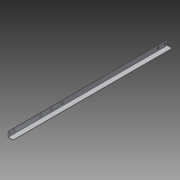
# Autodesk Inventor part: Shooter Side Support Bar - R
Saved by Autodesk Inventor 2014 SP1 (Build 180222100, 222)
## iProperties
Created: 2013-12-13
Part Number: Shooter Side Support Bar - R
Material: Aluminum 6061
Document SubType Name: Modeling
Designer: Moses
Mass: 32.4416 g
Surface Area: 311.167 cm^2
Volume: 11.9711 cm^3
Density: 2.71 g/cm^3
Appearance: Aluminum - Flat
Author: Moses
Autodesk Inventor part; units mm, degrees
ref_plane "YZ Plane" through (0, 0, 0) normal (1, 0, 0) x (0, 1, 0)
ref_plane "XZ Plane" through (0, 0, 0) normal (0, 1, 0) x (-1, 0, 0)
ref_plane "XY Plane" through (0, 0, 0) normal (0, 0, 1) x (1, 0, 0)
sketch "Sketch1" plane through (0, 0, 0) normal (0, 0, 1) x (1, 0, 0)
  line L0 (0, 0) -> (0, 15.875)
  line L1 (0, 15.875) -> (0.7937, 15.875)
  line L2 (0.7937, 15.875) -> (0.7938, 0.7937)
  line L3 (0.7938, 0.7937) -> (15.875, 0.7937)
  line L4 (15.875, 0.7937) -> (15.875, 0)
  line L5 (15.875, 0) -> (0, 0)
  dimension "d0" = 15.875
  dimension "d1" = 0.7937
  constraints: 12 end point, 3 horizontal, 3 vertical, 2 perpendicular
  measures "d0" distance of L0.start L0.end
  measures "d1" distance of L0.end L1.end
extrude "Extrusion1" add sketch "Sketch1" along normal blind 495.3
sketch "Sketch2" plane through (0, 0, 0) normal (-1, 0, 0) x (0, 0, 1)
  line L0 (276.0218, 396.0812) -> (276.0218, 91.2812) projected
  arc A0 (276.0218, 91.2812) -> (282.7782, 91.2812) centre (279.4, 91.2812) ccw projected
  line L1 (282.7782, 91.2812) -> (282.7782, 396.0812) projected
  arc A1 (282.7782, 396.0812) -> (276.0218, 396.0812) centre (279.4, 396.0812) ccw projected
  circle A2 centre (279.4, 27.7812) radius 3.3782 projected
  circle A3 centre (279.4, 59.5312) radius 3.3782 projected
  line L2 (292.1, 15.0812) -> (482.6, 15.0812) projected
  line L3 (482.6, 15.0812) -> (482.6, 484.9812) projected
  line L4 (482.6, 484.9812) -> (292.1, 484.9812) projected
  line L5 (292.1, 484.9812) -> (292.1, 15.0812) projected
  line L6 (149.0218, 396.0812) -> (149.0218, 91.2812) projected
  arc A4 (149.0218, 91.2812) -> (155.7782, 91.2812) centre (152.4, 91.2812) ccw projected
  line L7 (155.7782, 91.2812) -> (155.7782, 396.0812) projected
  arc A5 (155.7782, 396.0812) -> (149.0218, 396.0812) centre (152.4, 396.0812) ccw projected
  ellipse E0 centre (152.3984, 27.7812) end of major axis (152.3984, 31.1594) minor radius 3.3782 projected
  ellipse E1 centre (152.3984, 59.5312) end of major axis (152.3984, 56.153) minor radius 3.3782 projected
  line L8 (266.7, 15.0812) -> (266.7, 484.9812) projected
  line L9 (266.7, 484.9812) -> (165.1, 484.9812) projected
  line L10 (165.1, 484.9812) -> (165.1, 15.0812) projected
  line L11 (165.1, 15.0812) -> (266.7, 15.0812) projected
  line L12 (12.7, 15.0812) -> (139.7, 15.0812) projected
  line L13 (139.7, 15.0812) -> (139.7, 484.9812) projected
  line L14 (139.7, 484.9812) -> (12.7, 484.9812) projected
  line L15 (12.7, 484.9812) -> (12.7, 15.0812) projected
  circle A6 centre (393.7, 8.7312) radius 3.3782 projected
  circle A7 centre (393.7, 491.3312) radius 3.3782 projected
  circle A8 centre (405.6062, 8.7312) radius 3.3782 projected
  circle A9 centre (405.6062, 491.3312) radius 3.3782 projected
  circle A10 centre (417.5125, 8.7312) radius 3.3782 projected
  circle A11 centre (417.5125, 491.3312) radius 3.3782 projected
  circle A12 centre (429.4187, 8.7312) radius 3.3782 projected
  circle A13 centre (429.4187, 491.3312) radius 3.3782 projected
  circle A14 centre (441.325, 8.7312) radius 3.3782 projected
  circle A15 centre (441.325, 491.3312) radius 3.3782 projected
  circle A16 centre (453.2312, 8.7312) radius 3.3782 projected
  circle A17 centre (453.2312, 491.3312) radius 3.3782 projected
  circle A18 centre (465.1375, 8.7312) radius 3.3782 projected
  circle A19 centre (465.1375, 491.3312) radius 3.3782 projected
  circle A20 centre (477.0437, 8.7312) radius 3.3782 projected
  circle A21 centre (477.0437, 491.3312) radius 3.3782 projected
  circle A22 centre (382.6329, 8.7312) radius 3.3782 projected
  circle A23 centre (382.6329, 491.3312) radius 3.3782 projected
  circle A24 centre (371.5657, 8.7312) radius 3.3782 projected
  circle A25 centre (371.5657, 491.3312) radius 3.3782 projected
  circle A26 centre (360.4986, 8.7312) radius 3.3782 projected
  circle A27 centre (360.4986, 491.3312) radius 3.3782 projected
  circle A28 centre (349.4314, 8.7312) radius 3.3782 projected
  circle A29 centre (349.4314, 491.3312) radius 3.3782 projected
  circle A30 centre (338.3643, 8.7312) radius 3.3782 projected
  circle A31 centre (338.3643, 491.3312) radius 3.3782 projected
  circle A32 centre (327.2971, 8.7312) radius 3.3782 projected
  circle A33 centre (327.2971, 491.3312) radius 3.3782 projected
  circle A34 centre (316.23, 8.7312) radius 3.3782 projected
  circle A35 centre (316.23, 491.3312) radius 3.3782 projected
  circle A36 centre (305.1629, 8.7312) radius 3.3782 projected
  circle A37 centre (305.1629, 491.3312) radius 3.3782 projected
  circle A38 centre (294.0957, 8.7312) radius 3.3782 projected
  circle A39 centre (294.0957, 491.3312) radius 3.3782 projected
  circle A40 centre (283.0286, 8.7312) radius 3.3782 projected
  circle A41 centre (283.0286, 491.3312) radius 3.3782 projected
  circle A42 centre (271.9614, 8.7312) radius 3.3782 projected
  circle A43 centre (271.9614, 491.3312) radius 3.3782 projected
  circle A44 centre (260.8943, 8.7312) radius 3.3782 projected
  circle A45 centre (260.8943, 491.3312) radius 3.3782 projected
  circle A46 centre (249.8271, 8.7312) radius 3.3782 projected
  circle A47 centre (249.8271, 491.3312) radius 3.3782 projected
  circle A48 centre (238.76, 8.7312) radius 3.3782 projected
  circle A49 centre (238.76, 491.3312) radius 3.3782 projected
  circle A50 centre (227.6929, 8.7312) radius 3.3782 projected
  circle A51 centre (227.6929, 491.3312) radius 3.3782 projected
  circle A52 centre (216.6257, 8.7312) radius 3.3782 projected
  circle A53 centre (216.6257, 491.3312) radius 3.3782 projected
  circle A54 centre (205.5586, 8.7312) radius 3.3782 projected
  circle A55 centre (205.5586, 491.3312) radius 3.3782 projected
  circle A56 centre (194.4914, 8.7312) radius 3.3782 projected
  circle A57 centre (194.4914, 491.3312) radius 3.3782 projected
  circle A58 centre (183.4243, 8.7312) radius 3.3782 projected
  circle A59 centre (183.4243, 491.3312) radius 3.3782 projected
  circle A60 centre (172.3571, 8.7312) radius 3.3782 projected
  circle A61 centre (172.3571, 491.3312) radius 3.3782 projected
  circle A62 centre (161.29, 8.7312) radius 3.3782 projected
  circle A63 centre (161.29, 491.3312) radius 3.3782 projected
  circle A64 centre (150.2229, 8.7312) radius 3.3782 projected
  circle A65 centre (150.2229, 491.3312) radius 3.3782 projected
  circle A66 centre (139.1557, 8.7312) radius 3.3782 projected
  circle A67 centre (139.1557, 491.3312) radius 3.3782 projected
  circle A68 centre (128.0886, 8.7312) radius 3.3782 projected
  circle A69 centre (128.0886, 491.3312) radius 3.3782 projected
  circle A70 centre (117.0214, 8.7312) radius 3.3782 projected
  circle A71 centre (117.0214, 491.3312) radius 3.3782 projected
  circle A72 centre (105.9543, 8.7312) radius 3.3782 projected
  circle A73 centre (105.9543, 491.3312) radius 3.3782 projected
  circle A74 centre (94.8871, 8.7312) radius 3.3782 projected
  circle A75 centre (94.8871, 491.3312) radius 3.3782 projected
  circle A76 centre (83.82, 8.7312) radius 3.3782 projected
  circle A77 centre (83.82, 491.3312) radius 3.3782 projected
  circle A78 centre (72.7529, 8.7312) radius 3.3782 projected
  circle A79 centre (72.7529, 491.3312) radius 3.3782 projected
  circle A80 centre (61.6857, 8.7312) radius 3.3782 projected
  circle A81 centre (61.6857, 491.3312) radius 3.3782 projected
  circle A82 centre (50.6186, 8.7312) radius 3.3782 projected
  circle A83 centre (50.6186, 491.3312) radius 3.3782 projected
  circle A84 centre (39.5514, 8.7312) radius 3.3782 projected
  circle A85 centre (39.5514, 491.3312) radius 3.3782 projected
  circle A86 centre (28.4843, 8.7312) radius 3.3782 projected
  circle A87 centre (28.4843, 491.3312) radius 3.3782 projected
  circle A88 centre (17.4171, 8.7312) radius 3.3782 projected
  circle A89 centre (17.4171, 491.3312) radius 3.3782 projected
  circle A90 centre (488.95, 8.7312) radius 3.3782 projected
  circle A91 centre (488.95, 18.5802) radius 3.3782 projected
  circle A92 centre (488.95, 28.4292) radius 3.3782 projected
  circle A93 centre (488.95, 38.2782) radius 3.3782 projected
  circle A94 centre (488.95, 48.1272) radius 3.3782 projected
  circle A95 centre (488.95, 57.9761) radius 3.3782 projected
  circle A96 centre (488.95, 67.8251) radius 3.3782 projected
  circle A97 centre (488.95, 77.6741) radius 3.3782 projected
  circle A98 centre (488.95, 87.5231) radius 3.3782 projected
  circle A99 centre (488.95, 97.3721) radius 3.3782 projected
  circle A100 centre (488.95, 107.221) radius 3.3782 projected
  circle A101 centre (488.95, 117.07) radius 3.3782 projected
  circle A102 centre (488.95, 126.919) radius 3.3782 projected
  circle A103 centre (488.95, 136.768) radius 3.3782 projected
  circle A104 centre (488.95, 146.617) radius 3.3782 projected
  circle A105 centre (488.95, 156.4659) radius 3.3782 projected
  circle A106 centre (488.95, 166.3149) radius 3.3782 projected
  circle A107 centre (488.95, 176.1639) radius 3.3782 projected
  circle A108 centre (488.95, 186.0129) radius 3.3782 projected
  circle A109 centre (488.95, 195.8619) radius 3.3782 projected
  circle A110 centre (488.95, 205.7108) radius 3.3782 projected
  circle A111 centre (488.95, 215.5598) radius 3.3782 projected
  circle A112 centre (488.95, 225.4088) radius 3.3782 projected
  circle A113 centre (488.95, 235.2578) radius 3.3782 projected
  circle A114 centre (488.95, 245.1068) radius 3.3782 projected
  circle A115 centre (488.95, 254.9557) radius 3.3782 projected
  circle A116 centre (488.95, 264.8047) radius 3.3782 projected
  circle A117 centre (488.95, 274.6537) radius 3.3782 projected
  circle A118 centre (488.95, 284.5027) radius 3.3782 projected
  circle A119 centre (488.95, 294.3517) radius 3.3782 projected
  circle A120 centre (488.95, 304.2006) radius 3.3782 projected
  circle A121 centre (488.95, 314.0496) radius 3.3782 projected
  circle A122 centre (488.95, 323.8986) radius 3.3782 projected
  circle A123 centre (488.95, 333.7476) radius 3.3782 projected
  circle A124 centre (488.95, 343.5966) radius 3.3782 projected
  circle A125 centre (488.95, 353.4455) radius 3.3782 projected
  circle A126 centre (488.95, 363.2945) radius 3.3782 projected
  circle A127 centre (488.95, 373.1435) radius 3.3782 projected
  circle A128 centre (488.95, 382.9925) radius 3.3782 projected
  circle A129 centre (488.95, 392.8415) radius 3.3782 projected
  circle A130 centre (488.95, 402.6904) radius 3.3782 projected
  circle A131 centre (488.95, 412.5394) radius 3.3782 projected
  circle A132 centre (488.95, 422.3884) radius 3.3782 projected
  circle A133 centre (488.95, 432.2374) radius 3.3782 projected
  circle A134 centre (488.95, 442.0864) radius 3.3782 projected
  circle A135 centre (488.95, 451.9353) radius 3.3782 projected
  circle A136 centre (488.95, 461.7843) radius 3.3782 projected
  circle A137 centre (488.95, 471.6333) radius 3.3782 projected
  circle A138 centre (488.95, 481.4823) radius 3.3782 projected
  circle A139 centre (488.95, 491.3312) radius 3.3782 projected
  circle A140 centre (6.35, 8.7312) radius 3.3782 projected
  circle A141 centre (6.35, 18.5802) radius 3.3782 projected
  circle A142 centre (6.35, 28.4292) radius 3.3782 projected
  circle A143 centre (6.35, 38.2782) radius 3.3782 projected
  circle A144 centre (6.35, 48.1272) radius 3.3782 projected
  circle A145 centre (6.35, 57.9761) radius 3.3782 projected
  circle A146 centre (6.35, 67.8251) radius 3.3782 projected
  circle A147 centre (6.35, 77.6741) radius 3.3782 projected
  circle A148 centre (6.35, 87.5231) radius 3.3782 projected
  circle A149 centre (6.35, 97.3721) radius 3.3782 projected
  circle A150 centre (6.35, 107.221) radius 3.3782 projected
  circle A151 centre (6.35, 117.07) radius 3.3782 projected
  circle A152 centre (6.35, 126.919) radius 3.3782 projected
  circle A153 centre (6.35, 136.768) radius 3.3782 projected
  circle A154 centre (6.35, 146.617) radius 3.3782 projected
  circle A155 centre (6.35, 156.4659) radius 3.3782 projected
  circle A156 centre (6.35, 166.3149) radius 3.3782 projected
  circle A157 centre (6.35, 176.1639) radius 3.3782 projected
  circle A158 centre (6.35, 186.0129) radius 3.3782 projected
  circle A159 centre (6.35, 195.8619) radius 3.3782 projected
  circle A160 centre (6.35, 205.7108) radius 3.3782 projected
  circle A161 centre (6.35, 215.5598) radius 3.3782 projected
  circle A162 centre (6.35, 225.4088) radius 3.3782 projected
  circle A163 centre (6.35, 235.2578) radius 3.3782 projected
  circle A164 centre (6.35, 245.1068) radius 3.3782 projected
  circle A165 centre (6.35, 254.9557) radius 3.3782 projected
  circle A166 centre (6.35, 264.8047) radius 3.3782 projected
  circle A167 centre (6.35, 274.6537) radius 3.3782 projected
  circle A168 centre (6.35, 284.5027) radius 3.3782 projected
  circle A169 centre (6.35, 294.3517) radius 3.3782 projected
  circle A170 centre (6.35, 304.2006) radius 3.3782 projected
  circle A171 centre (6.35, 314.0496) radius 3.3782 projected
  circle A172 centre (6.35, 323.8986) radius 3.3782 projected
  circle A173 centre (6.35, 333.7476) radius 3.3782 projected
  circle A174 centre (6.35, 343.5966) radius 3.3782 projected
  circle A175 centre (6.35, 353.4455) radius 3.3782 projected
  circle A176 centre (6.35, 363.2945) radius 3.3782 projected
  circle A177 centre (6.35, 373.1435) radius 3.3782 projected
  circle A178 centre (6.35, 382.9925) radius 3.3782 projected
  circle A179 centre (6.35, 392.8415) radius 3.3782 projected
  circle A180 centre (6.35, 402.6904) radius 3.3782 projected
  circle A181 centre (6.35, 412.5394) radius 3.3782 projected
  circle A182 centre (6.35, 422.3884) radius 3.3782 projected
  circle A183 centre (6.35, 432.2374) radius 3.3782 projected
  circle A184 centre (6.35, 442.0864) radius 3.3782 projected
  circle A185 centre (6.35, 451.9353) radius 3.3782 projected
  circle A186 centre (6.35, 461.7843) radius 3.3782 projected
  circle A187 centre (6.35, 471.6333) radius 3.3782 projected
  circle A188 centre (6.35, 481.4823) radius 3.3782 projected
  circle A189 centre (6.35, 491.3312) radius 3.3782 projected
  line L16 (0, 2.3812) -> (0, 497.6812) projected
  line L17 (0, 497.6812) -> (495.3, 497.6812) projected
  line L18 (495.3, 497.6812) -> (495.3, 2.3812) projected
  line L19 (495.3, 2.3812) -> (0, 2.3812) projected
  constraints: 2 other
extrude "Extrusion2" cut sketch "Sketch2" against normal through all contours A6 | A20 | A26 | A32 | A86 | A90 | A140
body "Solid1"
